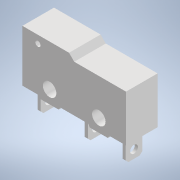
# Autodesk Inventor part: Body
Saved by Autodesk Inventor 2023 (Build 270158000, 158)
## iProperties
Created: 2019-04-17
Part Number: Body
Material: Generic
Document SubType Name: Modeling
Designer: Parker
Density: 1 g/cm^3
Appearance: Default
Author: Parker
Autodesk Inventor part; units mm, degrees
ref_plane "YZ Plane" through (0, 0, 0) normal (1, 0, 0) x (0, 1, 0)
ref_plane "XZ Plane" through (0, 0, 0) normal (0, 1, 0) x (-1, 0, 0)
ref_plane "XY Plane" through (0, 0, 0) normal (0, 0, 1) x (1, 0, 0)
sketch "Sketch1" plane through (0, 0, 0) normal (0, 0, 1) x (1, 0, 0)
  line L0 (-10, 5) -> (10, 5)
  line L1 (10, 5) -> (10, -5)
  line L2 (10, -5) -> (-10, -5)
  line L3 (-10, -5) -> (-10, 5)
  point P0 (0, 0)
  dimension "d0" = 20
  dimension "d1" = 10
  dimension "d2" = 10
  dimension "d3" = 5
  constraints: 8 end point, 2 parallel, 1 horizontal, 1 perpendicular
  measures "d0" distance of L0.start L0.end
  measures "d1" distance from line of L3 point (0, 0)
  measures "d2" distance of L2.end L0.start
  measures "d3" distance from line of point (0, 0) L2
extrude "Extrusion1" add sketch "Sketch1" along normal blind 6.1
sketch "Sketch2" plane through (0, 0, 6.1) normal (0, 0, 1) x (1, 0, 0)
  line L0 (10, 5) -> (-10, 5) projected
  line L1 (-1, 5) -> (0, 4)
  line L2 (0, 4) -> (10, 4)
  line L3 (10, -5) -> (10, 5) projected
  line L4 (10, 5) -> (10, 4)
  line L5 (-1, 5) -> (10, 5)
  point P0 (0, 0)
  dimension "d6" = 10
  dimension "d7" = 1
  dimension "d8" = 1
  constraints: 8 end point, 2 point on line, 1 collinear, 1 horizontal, 1 perpendicular
  measures "d6" distance of L1.end L2.end
  measures "d7" horizontal distance of L1.end L1.start
  measures "d8" distance between parallel lines of L0 L2
extrude "Extrusion2" cut sketch "Sketch2" against normal through all
sketch "Sketch3" plane through (0, 0, 6.1) normal (0, 0, 1) x (1, 0, 0)
  line L0 (-10, 5) -> (-10, -5) projected
  line L1 (10, -5) -> (10, 4) projected
  line L2 (-10, -5) -> (10, -5) projected
  point P0 (0, 0)
  point P1 (-4.75, -3)
  point P2 (4.75, -3)
  dimension "d36" = 5.25
  dimension "d38" = 2
  dimension "d39" = 2
  dimension "d41" = 9.5
  measures "d36" distance from line of L0 point (-4.75, -3)
  measures "d38" distance from line of L2 point (-4.75, -3)
  measures "d39" distance from line of L2 point (4.75, -3)
  measures "d41" distance of point (4.75, -3) point (-4.75, -3)
sketch "Sketch4" plane through (0, 0, 6.1) normal (0, 0, 1) x (1, 0, 0)
  line L0 (-10, -5) -> (10, -5) projected
  line L1 (-10, 5) -> (-10, -5) projected
  line L2 (-6.75, -5) -> (-6.5, -5.5)
  line L3 (-6.5, -5.5) -> (-3, -5.5)
  line L4 (-3, -5.5) -> (-2.75, -5)
  line L5 (-6.75, -5) -> (-2.75, -5)
  line L6 (2.75, -5) -> (3, -5.5)
  line L7 (3, -5.5) -> (6.5, -5.5)
  line L8 (6.5, -5.5) -> (6.75, -5)
  line L9 (2.75, -5) -> (6.75, -5)
  line L10 (10, -5) -> (10, 4) projected
  point P0 (0, 0)
  point P1 (6.75, -5)
  dimension "d16" = 0.5
  dimension "d17" = 4
  dimension "d19" = 3.5
  dimension "d20" = 0.25
  dimension "d22" = 4
  dimension "d23" = 3.5
  dimension "d24" = 0.25
  dimension "d25" = 0.5
  dimension "d26" = 0
  dimension "d40" = 3.5
  dimension "d43" = 3.5
  constraints: 16 end point, 3 point on line, 2 horizontal, 1 collinear
  measures "d16" distance between parallel lines of L0 L3
  measures "d17" distance of L4.end L2.start
  measures "d19" distance of L2.end L3.end
  measures "d20" horizontal distance of L2.start L2.end
  measures "d22" distance of L6.start L8.end
  measures "d23" distance of L6.end L7.end
  measures "d24" horizontal distance of L6.start L6.end
  measures "d25" distance between parallel lines of L0 L7
  measures "d26" distance between parallel lines of L0 L9
  measures "d40" distance from line of L1 L2.end
  measures "d43" distance from line of L10 L7.end
extrude "Extrusion3" add sketch "Sketch4" against normal blind 6.1
hole "Hole1" at (-4.75, -3, 6.1) at (4.75, -3, 6.1) direction (0, 0, -1) diameter 2.6 end through all
sketch "Sketch5" plane through (-2.75, -5, 0) normal (0, -1, 0) x (1, 0, 0)
  line L0 (-7.25, 0) -> (-7.25, 6.1) projected
  line L1 (-7.25, 3.05) -> (12.75, 3.05)
  line L2 (12.75, 0) -> (12.75, 6.1) projected
  line L3 (-5.15, 1.45) -> (-5.75, 1.45)
  line L4 (-5.75, 1.45) -> (-5.75, 4.65)
  line L5 (-5.75, 4.65) -> (-5.15, 4.65)
  line L6 (-5.15, 4.65) -> (-5.15, 1.45)
  line L7 (-5.15, 1.45) -> (-5.75, 4.65) construction
  line L8 (-5.75, 1.45) -> (-5.15, 4.65) construction
  line L9 (3.95, 1.45) -> (3.35, 1.45)
  line L10 (3.35, 1.45) -> (3.35, 4.65)
  line L11 (3.35, 4.65) -> (3.95, 4.65)
  line L12 (3.95, 4.65) -> (3.95, 1.45)
  line L13 (3.95, 1.45) -> (3.35, 4.65) construction
  line L14 (3.35, 1.45) -> (3.95, 4.65) construction
  line L15 (11.25, 1.45) -> (10.65, 1.45)
  line L16 (10.65, 1.45) -> (10.65, 4.65)
  line L17 (10.65, 4.65) -> (11.25, 4.65)
  line L18 (11.25, 4.65) -> (11.25, 1.45)
  line L19 (11.25, 1.45) -> (10.65, 4.65) construction
  line L20 (10.65, 1.45) -> (11.25, 4.65) construction
  point P0 (2.75, 0)
  point P1 (-5.45, 3.05)
  point P2 (3.65, 3.05)
  point P3 (10.95, 3.05)
  dimension "d44" = 3.2
  dimension "d45" = 0.6
  dimension "d46" = 0.6
  dimension "d47" = 0.6
  dimension "d48" = 1.5
  dimension "d49" = 1.5
  dimension "d50" = 8.5
  constraints: 38 end point, 8 midpoint, 6 parallel, 5 point on line, 3 horizontal, 3 perpendicular
  measures "d44" distance of L15.end L16.end
  measures "d45" distance of L16.end L17.end
  measures "d46" distance of L10.end L11.end
  measures "d47" distance of L4.end L5.end
  measures "d48" distance between parallel lines of L2 L18
  measures "d49" distance between parallel lines of L0 L4
  measures "d50" distance between parallel lines of L10 L6
extrude "Extrusion4" add sketch "Sketch5" along normal blind 4.5
chamfer "Chamfer1" distance 0.5 angle 45 6 edges at (-8.2, -9.5, 4.65) (-8.2, -9.5, 1.45) (0.9, -9.5, 4.65) (0.9, -9.5, 1.45) (8.2, -9.5, 4.65) (8.2, -9.5, 1.45)
sketch "Sketch6" plane through (8.5, -5, 4.65) normal (1, 0, 0) x (0, 0, -1)
  line L0 (3.2, 0) -> (3.2, -4) projected
  line L1 (2.7, -4.5) -> (0.5, -4.5) projected
  point P0 (4.65, 5)
  point P1 (1.6, -2.9)
  dimension "d56" = 1.6
  dimension "d57" = 1.6
  measures "d56" distance from line of L0 point (1.6, -2.9)
  measures "d57" distance from line of L1 point (1.6, -2.9)
hole "Hole2" at (8.5, -7.9, 3.05) direction (-1, 0, 0) diameter 1.5 end through all
sketch "Sketch7" plane through (0, 0, 6.1) normal (0, 0, 1) x (1, 0, 0)
  line L0 (-10, 5) -> (-10, -5) projected
  line L1 (-1, 5) -> (-10, 5) projected
  point P0 (0, 0)
  point P1 (-7, 3.5)
  dimension "d65" = 3
  dimension "d66" = 1.5
  measures "d65" distance from line of L0 point (-7, 3.5)
  measures "d66" distance from line of L1 point (-7, 3.5)
hole "Hole3" at (-7, 3.5, 6.1) direction (0, 0, -1) diameter 1 end through all
body "Solid1"
